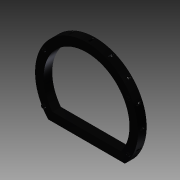
# Autodesk Inventor part: TSOP Ring
Saved by Autodesk Inventor 2015 (Build 190159000, 159)
## iProperties
Created: 2016-08-02
Part Number: TSOP Ring
Material: Generic
Document SubType Name: Modeling
Designer: James Yelland
Density: 1 g/cm^3
Appearance: Default
Author: James Yelland
Autodesk Inventor part; units mm, degrees
ref_plane "YZ Plane" through (0, 0, 0) normal (1, 0, 0) x (0, 1, 0)
ref_plane "XZ Plane" through (0, 0, 0) normal (0, 1, 0) x (-1, 0, 0)
ref_plane "XY Plane" through (0, 0, 0) normal (0, 0, 1) x (1, 0, 0)
sketch "Sketch1" plane through (0, 0, 0) normal (0, 1, 0) x (-1, 0, 0)
  circle A0 centre (73.6122, -42.5) radius 1.6
  circle A1 centre (73.6122, 42.5) radius 1.6
  circle A2 centre (-73.6122, 42.5) radius 1.6
  circle A3 centre (-73.6122, -42.5) radius 1.6
  line L0 (0, -60) -> (-67.082, -60)
  line L1 (0, -60) -> (67.082, -60)
  line L2 (0, -45) -> (60, -45)
  line L3 (0, -45) -> (-60, -45)
  arc A4 (60, -45) -> (-60, -45) centre (0, 0) ccw
  arc A5 (67.082, -60) -> (-67.082, -60) centre (0, 0) ccw
  line L4 (67.082, -60) -> (-67.082, -60)
  point P0 (0, 0)
  dimension "d4" = 3.2
  dimension "d5" = 3.2
  constraints: 10 end point, 6 centre point, 5 point on circle, 3 coincident, 2 point on line, 1 horizontal
  measures "d4" diameter of A0
  measures "d5" diameter of A1
extrude "Extrusion1" add sketch "Sketch1" along normal blind 15
sketch "Sketch2" plane through (0, 0, 0) normal (0, -1, 0) x (1, 0, 0)
  arc A0 (60, -45) -> (-60, -45) centre (0, 0) ccw projected
  line L0 (60, -45) -> (-60, -45) projected
  circle A1 centre (-73.6122, -42.5) radius 1.6 projected
  circle A2 centre (-73.6122, 42.5) radius 1.6 projected
  circle A3 centre (73.6122, 42.5) radius 1.6 projected
  circle A4 centre (73.6122, -42.5) radius 1.6 projected
  arc A5 (67.082, -60) -> (-67.082, -60) centre (0, 0) ccw projected
  line L1 (67.082, -60) -> (-67.082, -60) projected
  circle A6 centre (73.6122, 42.5) radius 3
  circle A7 centre (73.6122, -42.5) radius 1.6 projected
  circle A8 centre (73.6122, -42.5) radius 3
  circle A9 centre (-73.6122, -42.5) radius 1.6 projected
  circle A10 centre (-73.6122, -42.5) radius 3
  circle A11 centre (-73.6122, 42.5) radius 1.6 projected
  circle A12 centre (-73.6122, 42.5) radius 3
  point P0 (0, 0)
  dimension "d8" = 6
  dimension "d9" = 6
  dimension "d10" = 6
  dimension "d11" = 6
  constraints: 4 centre point, 4 coincident
  measures "d8" diameter of A6
  measures "d9" diameter of A8
  measures "d10" diameter of A10
  measures "d11" diameter of A12
extrude "Extrusion2" add sketch "Sketch2" along normal blind 3 contours A6 | A8 | A10 | A12
sketch "Sketch3" plane through (0, 15, 0) normal (0, 1, 0) x (1, 0, 0)
  line L0 (-84.95, -5.4) -> (-80.15, -5.4)
  line L1 (-80.15, -5.4) -> (-80.15, 5.4)
  line L2 (-80.15, 5.4) -> (-84.95, 5.4)
  arc A0 (-84.95, 2.5807) -> (-84.95, -2.5807) centre (-84, 0) ccw
  line L3 (-84.95, -5.4) -> (-84.95, -2.5807)
  line L4 (-84.95, 2.5807) -> (-84.95, 5.4)
  line L5 (-86.75, 0) -> (-84, 0)
  line L6 (-84, 0) -> (-90, 0)
  line L7 (67.082, 60) -> (-67.082, 60)
  arc A1 (-67.082, 60) -> (67.082, 60) centre (0, 0) ccw
  line L8 (-80.5501, 27.52) -> (-76.1154, 25.6831)
  line L9 (-80.5501, 27.52) -> (-79.4712, 30.1247)
  line L10 (-77.6059, 32.1454) -> (-83.1492, 34.4415)
  line L11 (-80.1465, 33.1978) -> (-77.6059, 32.1454)
  arc A2 (-77.496, 34.8932) -> (-79.4712, 30.1247) centre (-77.6059, 32.1454) ccw
  line L12 (-76.1154, 25.6831) -> (-71.9825, 35.661)
  line L13 (-77.496, 34.8932) -> (-76.4171, 37.4979)
  line L14 (-71.9825, 35.661) -> (-76.4171, 37.4979)
  line L15 (-58.8333, 51.1965) -> (-55.4392, 47.8024)
  line L16 (-58.8333, 51.1965) -> (-56.8397, 53.1901)
  line L17 (-54.3431, 54.3431) -> (-58.5858, 58.5858)
  arc A3 (-53.1901, 56.8397) -> (-56.8397, 53.1901) centre (-54.3431, 54.3431) ccw
  line L18 (-55.4392, 47.8024) -> (-47.8024, 55.4392)
  line L19 (-53.1901, 56.8397) -> (-51.1965, 58.8333)
  line L20 (-47.8024, 55.4392) -> (-51.1965, 58.8333)
  line L21 (-27.9092, 53.2679) -> (-26.0723, 48.8333)
  line L22 (-27.9092, 53.2679) -> (-25.3045, 54.3468)
  line L23 (-22.5567, 54.4567) -> (-24.8528, 60)
  line L24 (-23.6091, 56.9974) -> (-22.5567, 54.4567)
  arc A4 (-20.536, 56.322) -> (-25.3045, 54.3468) centre (-22.5567, 54.4567) ccw
  line L25 (-26.0723, 48.8333) -> (-16.0944, 52.9663)
  line L26 (-20.536, 56.322) -> (-17.9313, 57.4009)
  line L27 (-16.0944, 52.9663) -> (-17.9313, 57.4009)
  line L28 (-5.4, 54.95) -> (-5.4, 50.15)
  line L29 (-5.4, 54.95) -> (-2.5807, 54.95)
  line L30 (0, 54) -> (0, 60)
  line L31 (0, 56.75) -> (0, 54)
  arc A5 (2.5807, 54.95) -> (-2.5807, 54.95) centre (0, 54) ccw
  line L32 (-5.4, 50.15) -> (5.4, 50.15)
  line L33 (2.5807, 54.95) -> (5.4, 54.95)
  line L34 (5.4, 50.15) -> (5.4, 54.95)
  line L35 (17.9313, 57.4009) -> (16.0944, 52.9663)
  line L36 (17.9313, 57.4009) -> (20.536, 56.322)
  line L37 (22.5567, 54.4567) -> (24.8528, 60)
  line L38 (23.6091, 56.9974) -> (22.5567, 54.4567)
  arc A6 (25.3045, 54.3468) -> (20.536, 56.322) centre (22.5567, 54.4567) ccw
  line L39 (16.0944, 52.9663) -> (26.0723, 48.8333)
  line L40 (25.3045, 54.3468) -> (27.9092, 53.2679)
  line L41 (26.0723, 48.8333) -> (27.9092, 53.2679)
  line L42 (51.1965, 58.8333) -> (47.8024, 55.4392)
  line L43 (51.1965, 58.8333) -> (53.1901, 56.8397)
  line L44 (54.3431, 54.3431) -> (58.5858, 58.5858)
  line L45 (56.2877, 56.2877) -> (54.3431, 54.3431)
  arc A7 (56.8397, 53.1901) -> (53.1901, 56.8397) centre (54.3431, 54.3431) ccw
  line L46 (47.8024, 55.4392) -> (55.4392, 47.8024)
  line L47 (56.8397, 53.1901) -> (58.8333, 51.1965)
  line L48 (55.4392, 47.8024) -> (58.8333, 51.1965)
  line L49 (76.4171, 37.4979) -> (71.9825, 35.661)
  line L50 (76.4171, 37.4979) -> (77.496, 34.8932)
  line L51 (77.6059, 32.1454) -> (83.1492, 34.4415)
  line L52 (80.1465, 33.1978) -> (77.6059, 32.1454)
  arc A8 (79.4712, 30.1247) -> (77.496, 34.8932) centre (77.6059, 32.1454) ccw
  line L53 (71.9825, 35.661) -> (76.1154, 25.6831)
  line L54 (79.4712, 30.1247) -> (80.5501, 27.52)
  line L55 (76.1154, 25.6831) -> (80.5501, 27.52)
  line L56 (84.95, 5.4) -> (80.15, 5.4)
  line L57 (84.95, 5.4) -> (84.95, 2.5807)
  line L58 (84, 0) -> (90, 0)
  line L59 (86.75, 0) -> (84, 0)
  arc A9 (84.95, -2.5807) -> (84.95, 2.5807) centre (84, 0) ccw
  line L60 (80.15, 5.4) -> (80.15, -5.4)
  line L61 (84.95, -2.5807) -> (84.95, -5.4)
  line L62 (80.15, -5.4) -> (84.95, -5.4)
  line L63 (80.5501, -27.52) -> (76.1154, -25.6831)
  line L64 (80.5501, -27.52) -> (79.4712, -30.1247)
  line L65 (77.6059, -32.1454) -> (83.1492, -34.4415)
  line L66 (80.1465, -33.1978) -> (77.6059, -32.1454)
  arc A10 (77.496, -34.8932) -> (79.4712, -30.1247) centre (77.6059, -32.1454) ccw
  line L67 (76.1154, -25.6831) -> (71.9825, -35.661)
  line L68 (77.496, -34.8932) -> (76.4171, -37.4979)
  line L69 (71.9825, -35.661) -> (76.4171, -37.4979)
  line L70 (63.8871, -56.2503) -> (60.493, -52.8562)
  line L71 (63.8871, -56.2503) -> (61.8935, -58.2439)
  line L72 (59.397, -59.397) -> (63.6396, -63.6396)
  line L73 (61.3415, -61.3415) -> (59.397, -59.397)
  arc A11 (58.2439, -61.8935) -> (61.8935, -58.2439) centre (59.397, -59.397) ccw
  line L74 (60.493, -52.8562) -> (52.8562, -60.493)
  line L75 (58.2439, -61.8935) -> (56.2503, -63.8871)
  line L76 (52.8562, -60.493) -> (56.2503, -63.8871)
  line L77 (37.4979, -76.4171) -> (35.661, -71.9825)
  line L78 (37.4979, -76.4171) -> (34.8932, -77.496)
  line L79 (32.1454, -77.6059) -> (34.4415, -83.1492)
  line L80 (33.1978, -80.1465) -> (32.1454, -77.6059)
  arc A12 (30.1247, -79.4712) -> (34.8932, -77.496) centre (32.1454, -77.6059) ccw
  line L81 (35.661, -71.9825) -> (25.6831, -76.1154)
  line L82 (30.1247, -79.4712) -> (27.52, -80.5501)
  line L83 (25.6831, -76.1154) -> (27.52, -80.5501)
  line L84 (5.4, -84.95) -> (5.4, -80.15)
  line L85 (5.4, -84.95) -> (2.5807, -84.95)
  line L86 (0, -84) -> (0, -90)
  line L87 (0, -86.75) -> (0, -84)
  arc A13 (-2.5807, -84.95) -> (2.5807, -84.95) centre (0, -84) ccw
  line L88 (5.4, -80.15) -> (-5.4, -80.15)
  line L89 (-2.5807, -84.95) -> (-5.4, -84.95)
  line L90 (-5.4, -80.15) -> (-5.4, -84.95)
  line L91 (-27.52, -80.5501) -> (-25.6831, -76.1154)
  line L92 (-27.52, -80.5501) -> (-30.1247, -79.4712)
  line L93 (-32.1454, -77.6059) -> (-34.4415, -83.1492)
  line L94 (-33.1978, -80.1465) -> (-32.1454, -77.6059)
  arc A14 (-34.8932, -77.496) -> (-30.1247, -79.4712) centre (-32.1454, -77.6059) ccw
  line L95 (-25.6831, -76.1154) -> (-35.661, -71.9825)
  line L96 (-34.8932, -77.496) -> (-37.4979, -76.4171)
  line L97 (-35.661, -71.9825) -> (-37.4979, -76.4171)
  line L98 (-56.2503, -63.8871) -> (-52.8562, -60.493)
  line L99 (-56.2503, -63.8871) -> (-58.2439, -61.8935)
  line L100 (-59.397, -59.397) -> (-63.6396, -63.6396)
  line L101 (-61.3415, -61.3415) -> (-59.397, -59.397)
  arc A15 (-61.8935, -58.2439) -> (-58.2439, -61.8935) centre (-59.397, -59.397) ccw
  line L102 (-52.8562, -60.493) -> (-60.493, -52.8562)
  line L103 (-61.8935, -58.2439) -> (-63.8871, -56.2503)
  line L104 (-60.493, -52.8562) -> (-63.8871, -56.2503)
  line L105 (-76.4171, -37.4979) -> (-71.9825, -35.661)
  line L106 (-76.4171, -37.4979) -> (-77.496, -34.8932)
  line L107 (-77.6059, -32.1454) -> (-83.1492, -34.4415)
  line L108 (-80.1465, -33.1978) -> (-77.6059, -32.1454)
  arc A16 (-79.4712, -30.1247) -> (-77.496, -34.8932) centre (-77.6059, -32.1454) ccw
  line L109 (-71.9825, -35.661) -> (-76.1154, -25.6831)
  line L110 (-79.4712, -30.1247) -> (-80.5501, -27.52)
  line L111 (-76.1154, -25.6831) -> (-80.5501, -27.52)
  line L112 (58.5858, 58.5858) -> (54.9462, 54.9462)
  line L113 (67.082, 60) -> (-67.082, 60) projected
  line L114 (-58.5858, 58.5858) -> (-54.9462, 54.9462)
  line L115 (60, 60) -> (58.5858, 58.5858)
  line L116 (-60, 60) -> (-58.5858, 58.5858)
  point P0 (0, 0)
  dimension "d22" = 360
  dimension "d14" = 5.4
  dimension "d15" = 4.8
  dimension "d16" = 10.8
  dimension "d17" = 2.75
  dimension "d18" = 1.8
  dimension "d19" = 6
  dimension "d24" = 2
  constraints: 232 end point, 35 point on circle, 17 centre point, 1 point on line, 1 other
  measures "d14" distance from line of L0 L6.start
  measures "d15" distance of L0.start L0.end
  measures "d16" distance of L0.end L1.end
  measures "d17" radius of A0
  measures "d18" horizontal distance of L5.start L0.start
  measures "d19" distance of L6.start L6.end
  measures "d24" distance of L115.start L115.end
extrude "Extrusion3" cut sketch "Sketch3" against normal blind 13 contours L3 A0 L4 L2 L1 L0 | L9 A2 L13 L14 L12 L8 | L16 A3 L19 L20 L18 L15 | L22 A4 L26 L27 L25 L21 | L29 A5 L33 L34 L32 L28 | L36 A6 L40 L41 L39 L35 | L43 A7 L47 L48 L46 L42 | L50 A8 L54 L55 L53 L49 | L57 A9 L61 L62 L60 L56 | L64 A10 L68 L69 L67 L63 | L71 A11 L75 L76 L74 L70 | L78 A12 L82 L83 L81 L77 | L85 A13 L89 L90 L88 L84 | L92 A14 L96 L97 L95 L91 | L99 A15 L103 L104 L102 L98 | L106 A16 L110 L111 L109 L105
sketch "Sketch4" plane through (76.1154, 2, -25.6831) normal (0.9238795, 0, -0.3826834) x (-0.3826834, 0, -0.9238795)
  line L0 (0, 13) -> (10.8, 13) projected
  line L1 (5.4, 13) -> (5.4, 3.5)
  line L2 (5.4, 3.5) -> (3.9, 3.5)
  line L3 (5.4, 3.5) -> (6.9, 3.5)
  arc A0 (3.9, 3.5) -> (6.9, 3.5) centre (5.4, 3.5) ccw
  line L4 (3.9, 3.5) -> (3.9, 8.5)
  line L5 (6.9, 3.5) -> (6.9, 8.5)
  line L6 (6.9, 8.5) -> (5.4, 8.5)
  arc A1 (6.9, 8.5) -> (3.9, 8.5) centre (5.4, 8.5) ccw
  point P0 (5.4, -2)
  dimension "d27" = 9.5
  dimension "d29" = 1.5
  dimension "d30" = 5
  constraints: 12 end point, 4 point on circle, 3 vertical, 2 centre point, 2 coincident, 2 horizontal, 1 midpoint, 1 perpendicular, 1 point on line
  measures "d27" distance of L1.start L1.end
  measures "d29" distance of L1.end L3.end
  measures "d30" distance of L2.end L4.end
extrude "Extrusion4" cut sketch "Sketch4" along normal blind 12
chamfer "Chamfer1" distance 0.5 angle 45 4 edges at (83.7116, 8, -33.0509) (83.1514, 12, -34.436) (82.5636, 8, -35.8225) (83.2194, 4.0113, -34.2715)
pattern_circular "Circular Pattern1" count 11 over 225 about axis through (0, -10, 0) along (0, -1, 0) of "Extrusion4", "Chamfer1"
sketch "Sketch5" plane through (55.4392, 2, -47.8024) normal (0.7071068, 0, -0.7071068) x (-0.7071068, 0, -0.7071068)
  line L0 (0, 13) -> (10.8, 13)
  line L1 (5.4, 13) -> (5.4, 3.5)
  line L2 (5.4, 3.5) -> (3.9, 3.5)
  line L3 (5.4, 3.5) -> (6.9, 3.5)
  arc A0 (3.9, 3.5) -> (6.9, 3.5) centre (5.4, 3.5) ccw
  line L4 (3.9, 3.5) -> (3.9, 8.5)
  line L5 (6.9, 3.5) -> (6.9, 8.5)
  line L6 (6.9, 8.5) -> (5.4, 8.5)
  arc A1 (6.9, 8.5) -> (3.9, 8.5) centre (5.4, 8.5) ccw
  point P0 (5.4, -2)
  point P1 (5.4, -2)
  dimension "d39" = 9.5
  dimension "d40" = 1.5
  dimension "d41" = 5
  constraints: 14 end point, 4 point on circle, 3 vertical, 2 centre point, 2 coincident, 2 horizontal, 1 midpoint, 1 perpendicular, 1 point on line
  measures "d39" distance of L1.start L1.end
  measures "d40" distance of L1.end L3.end
  measures "d41" distance of L2.end L4.end
extrude "Extrusion5" cut sketch "Sketch5" along normal blind 39.5
chamfer "Chamfer2" distance 0.5 angle 45 4 edges at (60, 12, -60) (57.8787, 8, -60) (60, 4, -60) (62.1213, 8, -60)
sketch "Sketch6" plane through (26.0723, 2, -48.8333) normal (0.3826834, 0, -0.9238795) x (-0.9238795, 0, -0.3826834)
  line L0 (0, 13) -> (10.8, 13)
  line L1 (5.4, 13) -> (5.4, 3.5)
  line L2 (5.4, 3.5) -> (3.9, 3.5)
  line L3 (5.4, 3.5) -> (6.9, 3.5)
  arc A0 (3.9, 3.5) -> (6.9, 3.5) centre (5.4, 3.5) ccw
  line L4 (3.9, 3.5) -> (3.9, 8.5)
  line L5 (6.9, 3.5) -> (6.9, 8.5)
  line L6 (6.9, 8.5) -> (5.4, 8.5)
  arc A1 (6.9, 8.5) -> (3.9, 8.5) centre (5.4, 8.5) ccw
  point P0 (5.4, -2)
  point P1 (5.4, -2)
  dimension "d47" = 9.5
  dimension "d48" = 1.5
  dimension "d49" = 5
  constraints: 14 end point, 4 point on circle, 3 vertical, 2 centre point, 2 coincident, 2 horizontal, 1 midpoint, 1 perpendicular, 1 point on line
  measures "d47" distance of L1.start L1.end
  measures "d48" distance of L1.end L3.end
  measures "d49" distance of L2.end L4.end
extrude "Extrusion6" cut sketch "Sketch6" along normal blind 12
chamfer "Chamfer3" distance 0.5 angle 45 4 edges at (24.8528, 12, -60) (23.2292, 8, -60) (24.8528, 4, -60) (26.4764, 8, -60)
sketch "Sketch7" plane through (5.4, 15, -50.15) normal (0, 0, -1) x (-1, 0, 0)
  line L0 (0, 0) -> (10.8, 0)
  line L1 (5.4, 0) -> (5.4, -9.5)
  line L2 (5.4, -9.5) -> (3.9, -9.5)
  line L3 (5.4, -9.5) -> (6.9, -9.5)
  arc A0 (3.9, -9.5) -> (6.9, -9.5) centre (5.4, -9.5) ccw
  line L4 (3.9, -9.5) -> (3.9, -4.5)
  line L5 (6.9, -9.5) -> (6.9, -4.5)
  line L6 (6.9, -4.5) -> (5.4, -4.5)
  arc A1 (6.9, -4.5) -> (3.9, -4.5) centre (5.4, -4.5) ccw
  point P0 (5.4, -15)
  point P1 (5.4, -2)
  dimension "d55" = 9.5
  dimension "d56" = 1.5
  dimension "d57" = 5
  constraints: 14 end point, 4 point on circle, 3 vertical, 2 centre point, 2 coincident, 2 horizontal, 1 midpoint, 1 perpendicular, 1 point on line
  measures "d55" distance of L1.start L1.end
  measures "d56" distance of L1.end L3.end
  measures "d57" distance of L2.end L4.end
extrude "Extrusion7" cut sketch "Sketch7" along normal blind 12
chamfer "Chamfer4" distance 0.5 angle 45 4 edges at (-1.5, 8, -60) (0, 4, -60) (1.5, 8, -60) (0, 12, -60)
fillet "Fillet1" radius 2 2 edges at (67.082, 7.5, -60) (-67.082, 7.5, -60)
sketch "Sketch8" plane through (-16.0944, 2, -52.9663) normal (-0.3826834, 0, -0.9238795) x (-0.9238795, 0, 0.3826834)
  line L0 (0, 13) -> (10.8, 13)
  line L1 (5.4, 13) -> (5.4, 3.5)
  line L2 (5.4, 3.5) -> (3.9, 3.5)
  line L3 (5.4, 3.5) -> (6.9, 3.5)
  arc A0 (3.9, 3.5) -> (6.9, 3.5) centre (5.4, 3.5) ccw
  line L4 (3.9, 3.5) -> (3.9, 8.5)
  line L5 (6.9, 3.5) -> (6.9, 8.5)
  line L6 (6.9, 8.5) -> (5.4, 8.5)
  arc A1 (6.9, 8.5) -> (3.9, 8.5) centre (5.4, 8.5) ccw
  point P0 (5.4, -2)
  point P1 (5.4, -2)
  dimension "d64" = 9.5
  dimension "d65" = 1.5
  dimension "d66" = 5
  constraints: 14 end point, 4 point on circle, 3 vertical, 2 centre point, 2 coincident, 2 horizontal, 1 midpoint, 1 perpendicular, 1 point on line
  measures "d64" distance of L1.start L1.end
  measures "d65" distance of L1.end L3.end
  measures "d66" distance of L2.end L4.end
extrude "Extrusion8" cut sketch "Sketch8" along normal blind 12
chamfer "Chamfer5" distance 0.5 angle 45 4 edges at (-26.4764, 8, -60) (-24.8528, 4, -60) (-23.2292, 8, -60) (-24.8528, 12, -60)
sketch "Sketch9" plane through (-47.8024, 2, -55.4392) normal (-0.7071068, 0, -0.7071068) x (-0.7071068, 0, 0.7071068)
  line L0 (0, 13) -> (10.8, 13)
  line L1 (5.4, 13) -> (5.4, 3.5)
  line L2 (5.4, 3.5) -> (3.9, 3.5)
  line L3 (5.4, 3.5) -> (6.9, 3.5)
  arc A0 (3.9, 3.5) -> (6.9, 3.5) centre (5.4, 3.5) ccw
  line L4 (3.9, 3.5) -> (3.9, 8.5)
  line L5 (6.9, 3.5) -> (6.9, 8.5)
  line L6 (6.9, 8.5) -> (5.4, 8.5)
  arc A1 (6.9, 8.5) -> (3.9, 8.5) centre (5.4, 8.5) ccw
  point P0 (5.4, -2)
  point P1 (5.4, -2)
  dimension "d72" = 9.5
  dimension "d73" = 1.5
  dimension "d74" = 5
  constraints: 14 end point, 4 point on circle, 3 vertical, 2 centre point, 2 coincident, 2 horizontal, 1 midpoint, 1 perpendicular, 1 point on line
  measures "d72" distance of L1.start L1.end
  measures "d73" distance of L1.end L3.end
  measures "d74" distance of L2.end L4.end
extrude "Extrusion9" cut sketch "Sketch9" along normal blind 34
chamfer "Chamfer6" distance 0.5 angle 45 4 edges at (-60, 12, -60) (-62.1213, 8, -60) (-60, 4, -60) (-57.8787, 8, -60)
body "Solid1"
